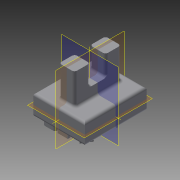
# Autodesk Inventor part: ChassisRechtsUntenKlappeSchluesselKopf
Saved by Autodesk Inventor 2015 (Build 190159000, 159)
## iProperties
Created: 2018-12-06
Part Number: ChassisRechtsUntenKlappeSchluesselKopf
Material: Generisch
Document SubType Name: Modeling
Designer: Boris
Density: 1 g/cm^3
Appearance: Vorgabe
Author: Boris
Autodesk Inventor part; units mm, degrees
sketch "Skizze1" plane through (0, 0, 0) normal (0, 0, 1) x (1, 0, 0)
  line L0 (-2.5, 3) -> (2.5, 3)
  line L1 (2.5, 3) -> (2.5, -3)
  line L2 (2.5, -3) -> (-2.5, -3)
  line L3 (-2.5, -3) -> (-2.5, 3)
  line L4 (0, 4.2) -> (0, -4.2) projected
  line L5 (-3.5, 0) -> (3.5, 0) projected
  point P0 (0, 0)
  dimension "d0" = 6
  dimension "d1" = 5
  constraints: 8 end point, 2 parallel, 1 horizontal, 1 perpendicular, 2 other
  measures "d0" distance of L0.end L1.end
  measures "d1" distance of L1.end L2.end
extrude "Extrusion1" add sketch "Skizze1" along normal mid plane 2
sketch "Skizze2" plane through (0, 0, 1) normal (0, 0, 1) x (1, 0, 0)
  line L0 (-0.75, 2.25) -> (0.75, 2.25)
  line L1 (0.75, 2.25) -> (0.75, 0.75)
  line L2 (0.75, 0.75) -> (-0.75, 0.75)
  line L3 (-0.75, 0.75) -> (-0.75, 2.25)
  line L4 (0, 4.2) -> (0, -4.2) projected
  line L5 (-3.5, 0) -> (3.5, 0) projected
  line L6 (-0.75, -2.25) -> (0.75, -2.25)
  line L7 (0.75, -2.25) -> (0.75, -0.75)
  line L8 (0.75, -0.75) -> (-0.75, -0.75)
  line L9 (-0.75, -0.75) -> (-0.75, -2.25)
  point P0 (0, 0)
  dimension "d4" = 1.5
  dimension "d5" = 1.5
  dimension "d6" = 0.75
  constraints: 16 end point, 4 symmetric about line, 2 parallel, 1 horizontal, 1 perpendicular, 1 other
  measures "d4" distance of L1.end L2.end
  measures "d5" distance of L0.end L1.end
  measures "d6" distance between parallel lines of L5 L2
extrude "Extrusion2" add sketch "Skizze2" along normal blind 3
sketch "Skizze3" plane through (0, 0, 1) normal (0, 0, 1) x (1, 0, 0)
  line L0 (0.75, 0.75) -> (-0.75, 0.75) projected
  line L1 (-0.75, -0.75) -> (0.75, -0.75) projected
  line L2 (-0.75, 0.75) -> (-0.75, -0.75)
  line L3 (0.75, 0.75) -> (0.75, -0.75)
  line L4 (0.75, -0.75) -> (0.75, -2.25) projected
  point P0 (0, 0)
  constraints: 4 end point, 1 collinear, 1 vertical
extrude "Extrusion3" add sketch "Skizze3" along normal blind 1
fillet "Rundung1" radius 0.25 8 edges at (-0.75, 2.25, 2.5) (0.75, 2.25, 2.5) (0.75, 0.75, 3) (-0.75, 0.75, 3) (-0.75, -0.75, 3) (0.75, -0.75, 3) (0.75, -2.25, 2.5) (-0.75, -2.25, 2.5)
fillet "Rundung2" radius 0.25 6 edges at (-0.6768, -0.8232, 2) (0.6768, -0.8232, 2) (0, -0.75, 2) (0.6768, 0.8232, 2) (-0.6768, 0.8232, 2) (0, 0.75, 2)
fillet "Rundung3" radius 0.25 8 edges at (-0.6768, 2.1768, 1) (0, 2.25, 1) (0.6768, 2.1768, 1) (0.75, 0, 1) (0.6768, -2.1768, 1) (0, -2.25, 1) (-0.6768, -2.1768, 1) (-0.75, 0, 1)
sketch "Skizze4" plane through (0, 0, -1) normal (0, 0, -1) x (-1, 0, 0)
  line L0 (-1.5, -1.134) -> (-1, -2)
  line L1 (-1, -2) -> (-0.5, -1.134)
  line L2 (-1.5, -1.134) -> (-0.5, -1.134)
  line L3 (-2.5, -3) -> (2.5, -3) projected
  line L4 (-2.5, 3) -> (-2.5, -3) projected
  line L5 (-0.0342, -1.134) -> (0.9658, -1.134)
  line L6 (2.3987, -1.134) -> (2.3987, -1.9505)
  line L7 (2.1487, -2.2005) -> (1.4225, -2.2005)
  line L8 (1.1725, -1.9505) -> (1.1725, -1.134)
  line L9 (-0.0342, -1.3965) -> (0.5658, -1.3965)
  line L10 (0.5658, -1.3965) -> (-0.0342, -1.9248)
  line L11 (0.9658, -1.9248) -> (0.3658, -1.9248)
  line L12 (0.3658, -1.9248) -> (0.9658, -1.3965)
  arc A0 (0.5, -2.5) -> (1, -2) centre (0.5, -2) ccw projected
  line L13 (0.9658, -2.1818) -> (-0.0342, -2.1818)
  line L14 (0.9658, -1.134) -> (0.9658, -1.3965)
  line L15 (0.9658, -1.9248) -> (0.9658, -2.1818)
  line L16 (-0.0342, -2.1818) -> (-0.0342, -1.9248)
  line L17 (-0.0342, -1.3965) -> (-0.0342, -1.134)
  line L18 (2.0523, -1.134) -> (2.0523, -1.6748)
  line L19 (1.8023, -1.9248) -> (1.7628, -1.9248)
  line L20 (1.5128, -1.6748) -> (1.5128, -1.134)
  line L21 (1.1725, -1.134) -> (1.5128, -1.134)
  line L22 (2.0523, -1.134) -> (2.3987, -1.134)
  arc A1 (1.5128, -1.6748) -> (1.7628, -1.9248) centre (1.7628, -1.6748) ccw
  arc A2 (1.8023, -1.9248) -> (2.0523, -1.6748) centre (1.8023, -1.6748) ccw
  arc A3 (2.1487, -2.2005) -> (2.3987, -1.9505) centre (2.1487, -1.9505) ccw
  arc A4 (1.1725, -1.9505) -> (1.4225, -2.2005) centre (1.4225, -1.9505) ccw
  line L23 (3.5, 0) -> (-3.5, 0) projected
  line L24 (-1.5, 1.134) -> (-1, 2)
  line L25 (-1, 2) -> (-0.5, 1.134)
  line L26 (-1.5, 1.134) -> (-0.5, 1.134)
  point P0 (0, 0)
  dimension "d14" = 60
  dimension "d15" = 1
  dimension "d16" = 1.5
  dimension "d17" = 1
  dimension "d18" = 1
  dimension "d19" = 0.4
  dimension "d20" = 0.4
  dimension "d21" = 1
  dimension "d23" = 0.25
  constraints: 48 end point, 10 parallel, 9 point on circle, 8 perpendicular, 8 tangent, 5 horizontal, 4 centre point, 3 equal radius, 3 symmetric about line, 2 point on line
  measures "d14" angle of L1 L0
  measures "d15" distance from line of L3 L0.end
  measures "d16" distance from line of L4 L0.end
  measures "d17" distance of L0.start L1.end
  measures "d18" distance from line of L4 L0.start
  measures "d19" distance of L11.end L10.end
  measures "d20" distance of L12.end L9.end
  measures "d21" distance of L5.start L5.end
  measures "d23" radius of A1
extrude "Extrusion4" add sketch "Skizze4" along normal blind 1
fillet "Rundung4" radius 0.25 4 edges at (-2.5, 0, -1) (0, -3, -1) (2.5, 0, -1) (0, 3, -1)
fillet "Rundung5" radius 0.25 4 edges at (-2.5, 0, 1) (0, 3, 1) (2.5, 0, 1) (0, -3, 1)
